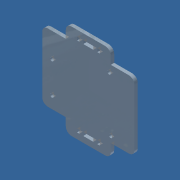
# Autodesk Inventor part: base2protopress
Saved by Autodesk Inventor 2014 (Build 180170000, 170)
## iProperties
Created: 2014-02-13
Part Number: base2protopress
Material: Generic
Document SubType Name: Modeling
Designer: Lefo
Density: 1 g/cm^3
Appearance: Clear
Author: Lefo
Autodesk Inventor part; units mm, degrees
ref_plane "YZ Plane" through (0, 0, 0) normal (1, 0, 0) x (0, 1, 0)
ref_plane "XZ Plane" through (0, 0, 0) normal (0, 1, 0) x (-1, 0, 0)
ref_plane "XY Plane" through (0, 0, 0) normal (0, 0, 1) x (1, 0, 0)
sketch "Sketch1" plane through (0, 0, 0) normal (0, 0, 1) x (1, 0, 0)
  line L0 (-28.2731, 30.1639) -> (-44.2731, 30.1639) projected
  arc A0 (11.7269, 37.1639) -> (6.7269, 42.1639) centre (6.7269, 37.1639) ccw projected
  line L1 (-23.2731, 42.1639) -> (6.7269, 42.1639) projected
  arc A1 (-23.2731, 42.1639) -> (-28.2731, 37.1639) centre (-23.2731, 37.1639) ccw projected
  line L2 (-28.2731, 30.1639) -> (-28.2731, 37.1639) projected
  line L3 (-28.2731, 30.1639) -> (-44.2731, 30.1639) projected
  arc A2 (-44.2731, 30.1639) -> (-49.2731, 25.1639) centre (-44.2731, 25.1639) ccw projected
  line L4 (-49.2731, 25.1639) -> (-49.2731, -25.1361) projected
  arc A3 (-49.2731, -25.1361) -> (-44.2731, -30.1361) centre (-44.2731, -25.1361) ccw projected
  line L5 (-44.2731, -30.1361) -> (-28.2731, -30.1361) projected
  line L6 (-28.2731, -30.1361) -> (-28.2731, -37.1361) projected
  arc A4 (-28.2731, -37.1361) -> (-23.2731, -42.1361) centre (-23.2731, -37.1361) ccw projected
  line L7 (-23.2731, -42.1361) -> (6.7269, -42.1361) projected
  arc A5 (6.7269, -42.1361) -> (11.7269, -37.1361) centre (6.7269, -37.1361) ccw projected
  line L8 (11.7269, -37.1361) -> (11.7269, -30.1361) projected
  line L9 (11.7269, -30.1361) -> (27.7269, -30.1361) projected
  arc A6 (27.7269, -30.1361) -> (32.7269, -25.1361) centre (27.7269, -25.1361) ccw projected
  line L10 (32.7269, -25.1361) -> (32.7269, 25.1639) projected
  arc A7 (32.7269, 25.1639) -> (27.7269, 30.1639) centre (27.7269, 25.1639) ccw projected
  line L11 (27.7269, 30.1639) -> (11.7269, 30.1639) projected
  line L12 (11.7269, 37.1639) -> (11.7269, 30.1639) projected
  line L13 (1.7269, 36.9139) -> (1.7269, 33.9139) projected
  line L14 (1.7269, 33.9139) -> (-0.2731, 33.9139) projected
  line L15 (-0.2731, 33.9139) -> (-0.2731, 36.9139) projected
  line L16 (-0.2731, 36.9139) -> (1.7269, 36.9139) projected
  line L17 (-16.2731, 36.9139) -> (-16.2731, 33.9139) projected
  line L18 (-16.2731, 33.9139) -> (-18.2731, 33.9139) projected
  line L19 (-18.2731, 33.9139) -> (-18.2731, 36.9139) projected
  line L20 (-18.2731, 36.9139) -> (-16.2731, 36.9139) projected
  line L21 (-3.7731, 36.9139) -> (-3.7731, 33.9139) projected
  line L22 (-3.7731, 33.9139) -> (-12.7731, 33.9139) projected
  line L23 (-12.7731, 33.9139) -> (-12.7731, 36.9139) projected
  line L24 (-12.7731, 36.9139) -> (-3.7731, 36.9139) projected
  line L25 (1.7269, -33.8861) -> (1.7269, -36.8861) projected
  line L26 (1.7269, -36.8861) -> (-0.2731, -36.8861) projected
  line L27 (-0.2731, -36.8861) -> (-0.2731, -33.8861) projected
  line L28 (-0.2731, -33.8861) -> (1.7269, -33.8861) projected
  line L29 (-16.2731, -33.8861) -> (-16.2731, -36.8861) projected
  line L30 (-16.2731, -36.8861) -> (-18.2731, -36.8861) projected
  line L31 (-18.2731, -36.8861) -> (-18.2731, -33.8861) projected
  line L32 (-18.2731, -33.8861) -> (-16.2731, -33.8861) projected
  line L33 (-3.7731, -33.8861) -> (-3.7731, -36.8861) projected
  line L34 (-3.7731, -36.8861) -> (-12.7731, -36.8861) projected
  line L35 (-12.7731, -36.8861) -> (-12.7731, -33.8861) projected
  line L36 (-12.7731, -33.8861) -> (-3.7731, -33.8861) projected
  circle A8 centre (10.1389, 23.4843) radius 1.6 projected
  circle A9 centre (-40.6611, 8.2443) radius 1.6 projected
  circle A10 centre (-40.6611, -19.6957) radius 1.6 projected
  circle A11 centre (11.4089, -24.7757) radius 1.6 projected
  point P0 (0, 0)
extrude "Extrusion1" add sketch "Sketch1" along normal blind 3
body "Solid1"
